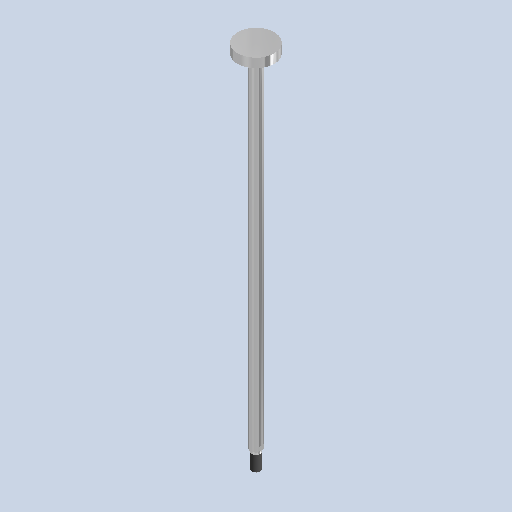
# Autodesk Inventor part: 193995 DSNU-63-500-P---(A---00--0-KS)
Saved by Autodesk Inventor 2025.2 (Build 292293000, 293)
## iProperties
Part Number: 193995 DSNU-63-500-P---(A---00--0-KS)
Material: Aluminum 6061
Catalog Web Link: www.cadenas.de
Description: DSNU---(KS)-Standard cylinder
Vendor: FESTO
Document SubType Name: Modeling
Designer: partserver
Manufacturer: FESTO
Mass: 645.271 g
Surface Area: 477.097 cm^2
Volume: 238.989 cm^3
Density: 2.7 g/cm^3
Appearance: Aluminum - Flat
Category: PARTsolutions
Company: FESTO
PSOL_IDENT_0: {$CADENAS_DATA\23d-libs\festo\parts\d\dsnu\parts\dsnu_metric_ks.prj},257 {VTYP=3D},{NB=193995 DSNU-6
PSOL_IDENT_1: 3-500-P---(A---00--0-KS)},{LINA=193995 DSNU-63-500-P},{NN=DSNU---(KS)},{DATE=01.06.2021 12:08:39},{G
PSOL_IDENT_2: EOMDATE=06.03.2020 09:03:14},{VERSION=},{LINEID=100},{WBVAR=TNR,HUB,DA,PE,ZD,VS,KA,K2A,K6,K3,K5,K8,K
PSOL_IDENT_3: P},{WBNUMERIC=HUB,K2A,K6,K8}  {NB=193995 DSNU-63-500-P---(A---00--0-KS)},{LINA=193995 DSNU-63-500-P}
PSOL_IDENT_4: ,{KT=DUMMY},{TNR=193995},{TYP=DSNU-63},{DSNU=METRIC},{KDM=63},{HUB=500},{DA=P},{DA1='P','PPV','PPS'}
PSOL_IDENT_5: ,{PE=A},{ZD=-},{VS=-},{VSALG='-','Q'},{KA=-},{KAALG='-','S2'},{K2A=0},{K6=0},{K3=-},{K31='-','K3'},{
PSOL_IDENT_6: K5=-},{K51='-','M16'},{K8=0},{KP=-},{KPALG='-','KP'},{A1=70},{A2=500},{A3=10},{A4=87.5},{AB=44},{AM=
PSOL_IDENT_7: 32},{B=45},{BB=4},{BE=M45x1,5},{BENDM=45.000},{BEKDM=43.160},{BEP=1.500},{BS=11.0},{B1=72},{B2=17},{
PSOL_IDENT_8: B3=44},{B4=15},{B5=36.0},{B6=18},{B7=4},{CD=16},{D=70},{D1=45},{D2=20},{D3=65.4},{D4=16.0},{D5=66.0}
PSOL_IDENT_9: ,{D6=60},{D7=45},{EE=G3/8},{EENDM=16.662},{EEKDM=14.950},{EW=21},{F=52},{FF=M8},{FFNDM=8.000},{FFKDM=
PSOL_IDENT_10: 6.466},{F1=36},{H=72},{H1=8},{KK=M16x1.5},{KKNDM=16.000},{KKKDM=0.000},{KKP=1.500},{K1=M10},{K1NDM=1
PSOL_IDENT_11: 0.000},{K1KDM=8.160},{K2=3.5},{KV=0},{KW=10},{L=16},{LH=15.0},{LK=28.0},{L1=172.2},{L2=94.2},{L3=13.
PSOL_IDENT_12: 0},{L4=33.0},{L5=30},{L6=77},{L7=44},{L8=28.0},{L9=32.0},{L10=117.2},{L11=132.2},{L12=94.2},{L13=184
PSOL_IDENT_13: .2},{ST=11.0},{SW=17},{T=16},{WH=45},{X=4.7},{XC=156.2},{K1KP=72},{K2KP=M10},{K2KPNDM=10.000},{K3KP=
PSOL_IDENT_14: 21},{K4KP=36.0},{K5KP=121.5},{K6KP=8.5},{K7KP=38},{K8KP=54.0},{K9KP=24.0},{K10KP=8.0},{K11KP=32},{K1
PSOL_IDENT_15: 2KP=G1/8},{K12KPNDM=9.728},{K13KP=86},{ZRSTART=61},{MHL=51.000},{ZRL=38.2},{C=25.200},{WHX=15.000},{
PSOL_IDENT_16: LD1=42.800},{LD2=42.800},{AD1=17.000},{AD2=13.000},{AD3=17.000},{AD4=13.000},{AD5=13.000},{MH1=14.00
PSOL_IDENT_17: 0},{MH2=3.100},{MH3=20.200},{KP1=48.000},{KP2=33.000},{KP3=25.000},{KP4=40.000},{KP5=50.000},{KPC=36
PSOL_IDENT_18: .000},{KPF=3.000},{KPG=30.000},{KPH=115.500},{KPJ=37.500},{KPK=17.000},{KPL=6.000},{KPR3=1.500},{KPR=
PSOL_IDENT_19: 37.000},{KPS=28.500},{MLD1=62.000},{MLD2=58.000},{MLD3=5.000},{MLL1=18.000},{KL1=85.2},{KKC=13.9},{K
PSOL_IDENT_20: KD=2.6},{KKF=0.75},{SWL=8.000},{K3L=10.500},{HUB1=500},{FDTXF31=6.000},{FDTB31=8.000}
NB: 193995 DSNU-63-500-P---(A---00--0-KS)
NN: DSNU---(KS)
NT: Standard cylinder
NBSYN: $TNR. $TYP.-$HUB1.-$DA.---($PE.$ZD.$VS.$KA.$K2A.$K6.$K3.$K5.$K8.$KP.KS)
LINA: 193995 DSNU-63-500-P
CATALOG: Festo
TNR: 193995
TYP: DSNU-63
DSNU: METRIC
KDM: 63
HUB: 500
DA: P
DA1: 'P','PPV','PPS'
PE: A
ZD: -
VS: -
KA: -
K2A: 0
K6: 0
K3: -
K31: '-','K3'
K5: -
K51: '-','M16'
K8: 0
KP: -
A1: 70
A2: 500
A3: 10
A4: 87.5
AB: 44
AM: 32
B: 45
BB: 4
BE: M45x1,5
BENDM: 45
BEKDM: 43.16
BEP: 1.5
BS: 11
B1: 72
B2: 17
B3: 44
B4: 15
B5: 36
B6: 18
B7: 4
CD: 16
D: 70
D1: 45
D2: 20
D3: 65.4
D4: 16
D5: 66
D6: 60
D7: 45
EE: G3/8
EENDM: 16.662
EEKDM: 14.95
EW: 21
F: 52
FF: M8
FFNDM: 8
FFKDM: 6.466
F1: 36
H: 72
H1: 8
KK: M16x1.5
KKNDM: 16
KKKDM: 0
KKP: 1.5
K1: M10
K1NDM: 10
K1KDM: 8.16
K2: 3.5
KV: 0
KW: 10
L: 16
LH: 15
LK: 28
L3: 13
L4: 33
L5: 30
L6: 77
L7: 44
L8: 28
L9: 32
L13: 184.2
ST: 11
SW: 17
T: 16
X: 4.7
K1KP: 72
K2KP: M10
K2KPNDM: 10
K3KP: 21
K4KP: 36
K5KP: 121.5
K6KP: 8.5
K7KP: 38
K8KP: 54
K9KP: 24
K10KP: 8
K11KP: 32
K12KP: G1/8
K12KPNDM: 9.728
K13KP: 86
MHL: 51
C: 25.2
WHX: 15
LD1: 42.8
LD2: 42.8
AD1: 17
AD2: 13
AD3: 17
AD4: 13
AD5: 13
MH1: 14
MH2: 3.1
MH3: 20.2
KP1: 48
KP2: 33
KP3: 25
KP4: 40
KP5: 50
KPC: 36
KPF: 3
KPG: 30
KPH: 115.5
KPJ: 37.5
KPK: 17
KPL: 6
KPR3: 1.5
KPR: 37
KPS: 28.5
MLD1: 62
MLD2: 58
MLD3: 5
MLL1: 18
SWL: 8
K3L: 10.5
FDTXF31: 6
FDTB31: 8
SUPPLIER: FESTO
ARTICLENO: 193995 DSNU-63-500-P---(A---00--0-KS)
BOMINFO: 193995 DSNU-63-500-P
CREATOR: CADENAS GmbH
Title: 193995 DSNU-63-500-P
Author: Cadenas PARTsolutions
Comments: Standard cylinder
Autodesk Inventor part; units mm, degrees
sketch "Sketch_2" plane through (0, 0, 0) normal (1, 0, 0) x (0, 1, 0)
  line L0 (0, -588.95) -> (0, 12)
  line L1 (0, 12) -> (10, 12)
  line L2 (10, 12) -> (10, -573.2)
  line L3 (10, -573.2) -> (31.5, -573.2)
  line L4 (31.5, -573.2) -> (31.5, -588.95)
  line L5 (31.5, -588.95) -> (0, -588.95)
  line L6 (0, -588.95) -> (0, 12)
  constraints: 14 end point
revolve "Revolution1" add sketch "Sketch_2" angle 360 about axis through (0, 0, -588.95) along (0, 0, -1)
sketch "Sketch_6" plane through (0, 0, 0) normal (1, 0, 0) x (0, 1, 0)
  line L0 (0, 11) -> (0, 44)
  line L1 (0, 44) -> (7.08, 44)
  line L2 (7.08, 44) -> (8, 43.08)
  line L3 (8, 43.08) -> (8, 17.4849)
  line L4 (8, 17.4849) -> (6.9952, 14.7243)
  arc A0 (6.9952, 14.7243) -> (6.95, 14.4678) centre (7.7, 14.4678) ccw
  line L5 (6.95, 14.4678) -> (6.95, 12.75)
  arc A1 (6.95, 12.75) -> (7.7, 12) centre (7.7, 12.75) ccw
  line L6 (7.7, 12) -> (8, 12)
  line L7 (8, 12) -> (8, 11)
  line L8 (8, 11) -> (0, 11)
  line L9 (0, 11) -> (0, 44)
  constraints: 20 end point, 4 point on circle, 2 centre point
revolve "Revolution2" add sketch "Sketch_6" angle 360 about axis through (0, 0, 11) along (0, 0, -1)
thread "Thread1" size "M16x1.5" class "6g" standard "ISO Metric profile" full length
sketch "Sketch_7" plane through (0, 0, 4) normal (0, 0, 1) x (1, 0, 0)
  line L0 (-17, 34) -> (-17, -17)
  line L1 (-17, -17) -> (-8.5, -17)
  line L2 (-8.5, -17) -> (-8.5, 17)
  line L3 (-8.5, 17) -> (8.5, 17)
  line L4 (8.5, 17) -> (8.5, -17)
  line L5 (8.5, -17) -> (17, -17)
  line L6 (17, -17) -> (17, 34)
  line L7 (17, 34) -> (-17, 34)
  constraints: 16 end point
extrude "Extrusion1" cut sketch "Sketch_7" along normal blind 9
ref_plane "FDT_KSAUFSATZ_XY" through (0, 0, 26) normal (0, 0, 1) x (-1, 0, 0)
ref_plane "FDT_KSAUFSATZ_YZ" through (0, 0, 26) normal (-1, 0, 0) x (0, -1, 0)
ref_plane "FDT_KSAUFSATZ_ZX" through (0, 0, 26) normal (0, -1, 0) x (0, 0, 1)
ref_plane "FDT_NUT_XY" through (0, 0, 26) normal (0, 0, 1) x (-1, 0, 0)
ref_plane "FDT_NUT_YZ" through (0, 0, 26) normal (-1, 0, 0) x (0, -1, 0)
ref_plane "FDT_NUT_ZX" through (0, 0, 26) normal (0, -1, 0) x (0, 0, 1)
ref_plane "KS_XY" through (0, 0, 0) normal (0, 0, -1) x (1, 0, 0)
ref_plane "KS_YZ" through (0, 0, 0) normal (1, 0, 0) x (0, -1, 0)
ref_plane "KS_ZX" through (0, 0, 0) normal (0, -1, 0) x (0, 0, -1)
ref_plane "NUT1_XY" through (0, 0, 32) normal (0, 0, 1) x (1, 0, 0)
ref_plane "NUT1_YZ" through (0, 0, 32) normal (1, 0, 0) x (0, 1, 0)
ref_plane "NUT1_ZX" through (0, 0, 32) normal (0, 1, 0) x (0, 0, 1)
body "Solid1"
